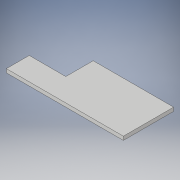
# Autodesk Inventor part: divider
Saved by Autodesk Inventor 2019 (Build 230136000, 136)
## iProperties
Created: 2018-06-15
Part Number: divider
Material: Generic
Document SubType Name: Modeling
Designer: daniel
Density: 1 g/cm^3
Appearance: Default
Author: daniel
Autodesk Inventor part; units mm, degrees
ref_plane "YZ Plane" through (0, 0, 0) normal (1, 0, 0) x (0, 1, 0)
ref_plane "XZ Plane" through (0, 0, 0) normal (0, 1, 0) x (-1, 0, 0)
ref_plane "XY Plane" through (0, 0, 0) normal (0, 0, 1) x (1, 0, 0)
sketch "Sketch2" plane through (0, 0, 0) normal (0, 0, 1) x (1, 0, 0)
  line L0 (-64, -2) -> (64, -2)
  line L1 (64, -2) -> (64, 2)
  line L2 (64, 2) -> (-64, 2)
  line L3 (-64, 2) -> (-64, -2)
  line L4 (-64, -2) -> (64, 2) construction
  line L5 (64, -2) -> (-64, 2) construction
  point P0 (0, 0)
  dimension "d0" = 4
  dimension "d1" = 128
  constraints: 12 end point, 2 midpoint, 2 parallel, 1 horizontal, 1 perpendicular
  measures "d0" distance of L1.end L0.end
  measures "d1" distance of L1.end L2.end
extrude "Extrusion1" add sketch "Sketch2" along normal blind 55
sketch "Sketch3" plane through (-64, -2, 0) normal (0, -1, 0) x (1, 0, 0)
  line L0 (0, 0) -> (128, 0) projected
  line L1 (0, 0) -> (40, 0)
  line L2 (40, 0) -> (40, 30)
  line L3 (40, 30) -> (0, 30)
  line L4 (0, 30) -> (0, 0)
  point P0 (64, 0)
  dimension "d4" = 40
  dimension "d5" = 30
  constraints: 8 end point, 2 parallel, 1 horizontal, 1 perpendicular
  measures "d4" distance of L3.end L2.end
  measures "d5" distance of L2.end L1.end
extrude "Extrusion2" cut sketch "Sketch3" against normal through all
body "Solid1"
